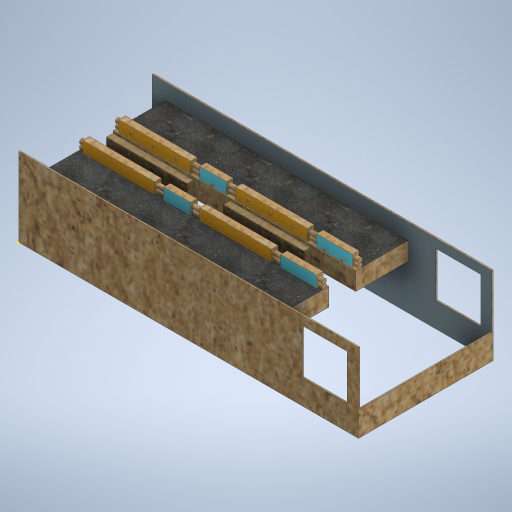
# Autodesk Inventor part: Walls
Saved by Autodesk Inventor 2024 (Build 280153000, 153)
## iProperties
Created: 2024-02-01
Part Number: Walls
Material: Generic
Document SubType Name: Modeling
Designer: HP
Density: 1 g/cm^3
Appearance: Default
Author: HP
Autodesk Inventor part; units mm, degrees
ref_plane "YZ Plane" through (0, 0, 0) normal (1, 0, 0) x (0, 1, 0)
sketch "Sketch2" plane through (0, 0, 0) normal (1, 0, 0) x (0, 1, 0)
  line L0 (0, 0) -> (175, 0)
  line L1 (175, 0) -> (175, 3)
  line L2 (175, 3) -> (0, 3)
  line L3 (0, 3) -> (0, 0)
  line L4 (0, 300) -> (175, 300)
  line L5 (175, 300) -> (175, 297)
  line L6 (175, 297) -> (0, 297)
  line L7 (0, 297) -> (0, 300)
  dimension "d8" = 175
  dimension "d9" = 3
  dimension "d10" = 175
  dimension "d11" = 3
  constraints: 16 end point, 4 parallel, 2 horizontal, 2 perpendicular, 1 point on line
  measures "d8" distance of L2.end L1.end
  measures "d9" distance of L1.end L0.end
  measures "d10" distance of L5.end L6.end
  measures "d11" distance of L4.end L5.end
extrude "Extrusion2" add sketch "Sketch2" along normal blind 756
sketch "Sketch3" plane through (0, 0, 300) normal (0, 0, 1) x (1, 0, 0)
  point P0 (0, 0)
sketch "Sketch4" plane through (0, 0, 300) normal (0, 0, 1) x (1, 0, 0)
  line L0 (0, 0) -> (3, 0)
  line L1 (3, 0) -> (3, 55)
  line L2 (3, 55) -> (0, 55)
  line L3 (0, 55) -> (0, 0)
  line L4 (756, 0) -> (753, 0)
  line L5 (753, 0) -> (753, 55)
  line L6 (753, 55) -> (756, 55)
  line L7 (756, 55) -> (756, 0)
  dimension "d30" = 100
  dimension "d31" = 100
  dimension "d32" = 25
  dimension "d41" = 55
  dimension "d14" = 3
  dimension "d15" = 55
  dimension "d16" = 3
  dimension "d17" = 55
  constraints: 16 end point, 4 parallel, 2 horizontal, 2 perpendicular
  measures "d14" distance of L2.end L1.end
  measures "d15" distance of L1.end L0.end
  measures "d16" distance of L5.end L6.end
  measures "d17" distance of L4.end L5.end
extrude "Extrusion3" add sketch "Sketch4" against normal through all
sketch "Sketch5" plane through (0, 0, 300) normal (0, 0, 1) x (1, 0, 0)
  point P0 (0, 0)
sketch "Sketch6" plane through (0, 0, 300) normal (0, 0, 1) x (1, 0, 0)
  point P0 (0, 0)
sketch "Sketch10" plane through (0, 0, 300) normal (0, 0, 1) x (1, 0, 0)
  line L0 (631, 155) -> (731, 155)
  line L1 (731, 155) -> (731, 55)
  line L2 (731, 55) -> (631, 55)
  line L3 (631, 55) -> (631, 155)
  line L4 (756, 175) -> (756, 0) projected
  line L5 (0, 175) -> (756, 175) projected
  line L6 (0, 0) -> (756, 0) projected
  dimension "d30" = 100
  dimension "d31" = 100
  dimension "d32" = 25
  dimension "d41" = 55
  constraints: 8 end point, 2 parallel, 1 horizontal, 1 perpendicular
  measures "d30" distance of L1.end L2.end
  measures "d31" distance of L0.end L1.end
  measures "d32" distance between parallel lines of L4 L1
  measures "d41" distance between parallel lines of L6 L2
extrude "Extrusion4" cut sketch "Sketch10" against normal through all
sketch "Sketch11" plane through (0, 0, 0) normal (0, -1, 0) x (1, 0, 0)
  point P0 (0, 0)
sketch "Sketch16" plane through (0, 0, 300) normal (0, 0, 1) x (1, 0, 0)
  line L0 (30, 140) -> (570, 140)
  line L1 (570, 140) -> (570, 100)
  line L2 (570, 100) -> (30, 100)
  line L3 (30, 100) -> (30, 140)
  line L4 (0, 175) -> (0, 0) projected
  line L5 (0, 0) -> (756, 0) projected
  point P0 (0, 87.5)
  dimension "d55" = 540
  dimension "d56" = 40
  dimension "d57" = 30
  dimension "d58" = 100
  constraints: 8 end point, 2 parallel, 1 horizontal, 1 midpoint, 1 perpendicular
  measures "d55" distance of L1.end L2.end
  measures "d56" distance of L0.end L1.end
  measures "d57" distance from line of point (0, 87.5) L3
  measures "d58" distance between parallel lines of L5 L2
extrude "Extrusion8" add sketch "Sketch16" against normal blind 120
ref_plane "Work Plane4" through (0, 0, 150) normal (0, 0, 1) x (1, 0, 0)
mirror "Mirror3" about plane through (0, 0, 150) normal (0, 0, 1) of "Extrusion8"
sketch "Sketch17" plane through (0, 0, 180) normal (0, 0, -1) x (-1, 0, 0)
  point P0 (0, 0)
sketch "Sketch19" plane through (0, 0, 180) normal (0, 0, -1) x (-1, 0, 0)
  line L0 (-210, 135) -> (-30, 135)
  line L1 (-30, 135) -> (-30, 105)
  line L2 (-30, 105) -> (-210, 105)
  line L3 (-210, 105) -> (-210, 135)
  line L4 (-570, 140) -> (-30, 140) projected
  line L5 (-30, 140) -> (-30, 100) projected
  point P0 (0, 0)
  dimension "d62" = 180
  dimension "d63" = 30
  dimension "d64" = 5
  dimension "d65" = 0
  constraints: 8 end point, 2 parallel, 1 horizontal, 1 perpendicular
  measures "d62" distance of L1.end L2.end
  measures "d63" distance of L0.end L1.end
  measures "d64" distance between parallel lines of L0 L4
  measures "d65" distance between parallel lines of L5 L1
extrude "Extrusion9" add sketch "Sketch19" along normal blind 15
sketch "Sketch21" plane through (0, 0, 165) normal (0, 0, -1) x (-1, 0, 0)
  circle A0 centre (-200, 127.5) radius 2.5
  line L0 (-210, 105) -> (-210, 135) projected
  line L1 (-210, 135) -> (-30, 135) projected
  circle A1 centre (-120, 127.5) radius 2.5
  circle A2 centre (-80, 127.5) radius 2.5
  circle A3 centre (-40, 127.5) radius 2.5
  line L2 (-30, 140) -> (-30, 100) projected
  circle A4 centre (-160, 127.5) radius 2.5
  line L3 (-30, 120) -> (-210, 120)
  circle A5 centre (-200, 112.5) radius 2.5
  circle A6 centre (-120, 112.5) radius 2.5
  circle A7 centre (-80, 112.5) radius 2.5
  circle A8 centre (-40, 112.5) radius 2.5
  circle A9 centre (-160, 112.5) radius 2.5
  point P0 (0, 0)
  dimension "d74" = 5
  dimension "d75" = 10
  dimension "d76" = 7.5
  dimension "d77" = 5
  dimension "d78" = 5
  dimension "d79" = 5
  dimension "d83" = 10
  dimension "d84" = 40
  dimension "d85" = 40
  dimension "d86" = 5
  dimension "d87" = 40
  dimension "d88" = 7.5
  dimension "d89" = 7.5
  dimension "d90" = 7.5
  dimension "d91" = 7.5
  constraints: 10 centre point, 5 symmetric about line, 2 end point, 2 midpoint, 5 other
  measures "d74" diameter of A0
  measures "d75" distance from line of L0 A0.centre
  measures "d76" distance from line of L1 A0.centre
  measures "d77" diameter of A1
  measures "d78" diameter of A2
  measures "d79" diameter of A3
  measures "d83" horizontal distance of L3.start A3.centre
  measures "d84" distance of A3.centre A2.centre
  measures "d85" distance of A2.centre A1.centre
  measures "d86" diameter of A4
  measures "d87" distance of A1.centre A4.centre
  measures "d88" distance from line of L1 A4.centre
  measures "d89" distance from line of L1 A1.centre
  measures "d90" distance from line of L1 A2.centre
  measures "d91" distance from line of L1 A3.centre
extrude "Extrusion11" cut sketch "Sketch21" against normal blind 3 contours A0 | A1 | A2 | A3 | A4 | A5 | A6 | A7 | A8 | A9
sketch "Sketch20" plane through (0, 0, 180) normal (0, 0, -1) x (-1, 0, 0)
  line L0 (-470, 135) -> (-290, 135)
  line L1 (-290, 135) -> (-290, 105)
  line L2 (-290, 105) -> (-470, 105)
  line L3 (-470, 105) -> (-470, 135)
  line L4 (-570, 140) -> (-30, 140) projected
  line L5 (-30, 140) -> (-30, 100) projected
  point P0 (0, 0)
  dimension "d68" = 180
  dimension "d69" = 30
  dimension "d70" = 5
  dimension "d71" = 260
  constraints: 8 end point, 2 parallel, 1 horizontal, 1 perpendicular
  measures "d68" distance of L1.end L2.end
  measures "d69" distance of L0.end L1.end
  measures "d70" distance between parallel lines of L4 L0
  measures "d71" distance between parallel lines of L5 L1
extrude "Extrusion10" add sketch "Sketch20" along normal blind 15
sketch "Sketch22" plane through (0, 0, 165) normal (0, 0, -1) x (-1, 0, 0)
  circle A0 centre (-460, 127.5) radius 2.5
  circle A1 centre (-420, 127.5) radius 2.5
  circle A2 centre (-380, 127.5) radius 2.5
  circle A3 centre (-340, 127.5) radius 2.5
  circle A4 centre (-300, 127.5) radius 2.5
  line L0 (-470, 135) -> (-290, 135) projected
  line L1 (-470, 105) -> (-470, 135) projected
  line L2 (-470, 120) -> (-290, 120)
  line L3 (-290, 135) -> (-290, 105) projected
  circle A5 centre (-460, 112.5) radius 2.5
  circle A6 centre (-420, 112.5) radius 2.5
  circle A7 centre (-380, 112.5) radius 2.5
  circle A8 centre (-340, 112.5) radius 2.5
  circle A9 centre (-300, 112.5) radius 2.5
  point P0 (0, 0)
  dimension "d94" = 5
  dimension "d95" = 5
  dimension "d96" = 5
  dimension "d97" = 5
  dimension "d98" = 5
  dimension "d99" = 7.5
  dimension "d100" = 7.5
  dimension "d101" = 7.5
  dimension "d102" = 7.5
  dimension "d103" = 10
  dimension "d104" = 40
  dimension "d105" = 40
  dimension "d106" = 40
  dimension "d107" = 40
  dimension "d108" = 7.5
  constraints: 10 centre point, 5 symmetric about line, 2 end point, 2 midpoint, 5 other
  measures "d94" diameter of A0
  measures "d95" diameter of A1
  measures "d96" diameter of A2
  measures "d97" diameter of A3
  measures "d98" diameter of A4
  measures "d99" distance from line of L0 A0.centre
  measures "d100" distance from line of L0 A1.centre
  measures "d101" distance from line of L0 A2.centre
  measures "d102" distance from line of L0 A3.centre
  measures "d103" distance from line of L1 A0.centre
  measures "d104" distance of A0.centre A1.centre
  measures "d105" distance of A1.centre A2.centre
  measures "d106" distance of A2.centre A3.centre
  measures "d107" distance of A4.centre A3.centre
  measures "d108" distance from line of L0 A4.centre
extrude "Extrusion12" cut sketch "Sketch22" against normal blind 3 contours A0 | A1 | A2 | A3 | A4 | A5 | A6 | A7 | A8 | A9
ref_plane "Work Plane5" through (0, 0, 150) normal (0, 0, 1) x (1, 0, 0)
mirror "Mirror4" about plane through (0, 0, 150) normal (0, 0, 1) of "Extrusion8", "Extrusion9", "Extrusion10", "Extrusion12", "Extrusion11"
sketch "Sketch23" plane through (570, 100, 3) normal (1, 0, 0) x (0, 0, -1)
  circle A0 centre (-107, 45) radius 5
  circle A1 centre (-107, 55) radius 5
  line L0 (0, 40) -> (-117, 40) projected
  line L1 (-117, 40) -> (-117, 0) projected
  point P0 (3, -100)
  point P1 (-107, 50)
  dimension "d112" = 10
  dimension "d113" = 10
  dimension "d114" = 5
  dimension "d115" = 10
  dimension "d116" = 0
  dimension "d117" = 10
  constraints: 2 centre point
  measures "d112" diameter of A0
  measures "d113" diameter of A1
  measures "d114" distance from line of L0 A0.centre
  measures "d115" distance of A0.centre A1.centre
  measures "d116" horizontal distance of A1.centre A0.centre
  measures "d117" distance from line of A0.centre L1
extrude "Extrusion13" add sketch "Sketch23" against normal blind 540
sketch "Sketch24" plane through (30, 140, 3) normal (0, 1, 0) x (1, 0, 0)
  line L0 (450, -114.5) -> (530, -114.5)
  line L1 (530, -114.5) -> (530, -99.5)
  line L2 (530, -99.5) -> (450, -99.5)
  line L3 (450, -99.5) -> (450, -114.5)
  line L4 (0, -117) -> (540, -117) projected
  line L5 (440, -117) -> (440, -132) projected
  point P0 (-30, 3)
  dimension "d120" = 80
  dimension "d121" = 15
  dimension "d122" = 2.5
  dimension "d123" = 10
  constraints: 8 end point, 2 parallel, 1 horizontal, 1 perpendicular
  measures "d120" distance of L2.end L1.end
  measures "d121" distance between parallel lines of L0 L2
  measures "d122" distance between parallel lines of L4 L0
  measures "d123" distance between parallel lines of L5 L3
extrude "Extrusion14" add sketch "Sketch24" along normal blind 25
sketch "Sketch25" plane through (30, 140, 3) normal (0, 1, 0) x (1, 0, 0)
  line L0 (270, -99.5) -> (430, -99.5)
  line L1 (430, -99.5) -> (430, -114.5)
  line L2 (430, -114.5) -> (270, -114.5)
  line L3 (270, -114.5) -> (270, -99.5)
  line L4 (0, -117) -> (540, -117) projected
  line L5 (260, -117) -> (260, -132) projected
  point P0 (-30, 3)
  dimension "d126" = 160
  dimension "d127" = 15
  dimension "d128" = 17.5
  dimension "d129" = 10
  constraints: 8 end point, 2 parallel, 1 horizontal, 1 perpendicular
  measures "d126" distance of L1.end L2.end
  measures "d127" distance of L0.end L1.end
  measures "d128" distance between parallel lines of L4 L0
  measures "d129" distance between parallel lines of L5 L3
extrude "Extrusion15" add sketch "Sketch25" along normal blind 25
sketch "Sketch26" plane through (30, 140, 3) normal (0, 1, 0) x (1, 0, 0)
  line L0 (190, -99.5) -> (250, -99.5)
  line L1 (250, -99.5) -> (250, -114.5)
  line L2 (250, -114.5) -> (190, -114.5)
  line L3 (190, -114.5) -> (190, -99.5)
  line L4 (0, -117) -> (540, -117) projected
  line L5 (180, -117) -> (180, -132) projected
  line L6 (10, -99.5) -> (170, -99.5)
  line L7 (170, -99.5) -> (170, -114.5)
  line L8 (170, -114.5) -> (10, -114.5)
  line L9 (10, -114.5) -> (10, -99.5)
  line L10 (0, -102) -> (0, -112) projected
  point P0 (-30, 3)
  point P1 (0, -107)
  dimension "d132" = 60
  dimension "d133" = 15
  dimension "d134" = 17.5
  dimension "d135" = 10
  dimension "d136" = 160
  dimension "d137" = 15
  dimension "d138" = 17.5
  dimension "d139" = 10
  constraints: 16 end point, 4 parallel, 2 horizontal, 2 perpendicular
  measures "d132" distance of L1.end L2.end
  measures "d133" distance of L0.end L1.end
  measures "d134" distance between parallel lines of L4 L0
  measures "d135" distance between parallel lines of L5 L3
  measures "d136" distance of L7.end L8.end
  measures "d137" distance of L6.end L7.end
  measures "d138" distance between parallel lines of L4 L6
  measures "d139" distance between parallel lines of L10 L9
extrude "Extrusion16" add sketch "Sketch26" along normal blind 25
sketch "Sketch27" plane through (480, 140, 117.5) normal (0, 0, 1) x (1, 0, 0)
  circle A0 centre (-50, 15) radius 2.5
  circle A1 centre (-100, 15) radius 2.5
  circle A2 centre (-150, 15) radius 2.5
  circle A3 centre (-310, 15) radius 2.5
  circle A4 centre (-360, 15) radius 2.5
  circle A5 centre (-410, 15) radius 2.5
  line L0 (-440, 20) -> (-440, 10) projected
  line L1 (-280, 10) -> (-280, 20) projected
  line L2 (-280, 25) -> (-440, 25) projected
  line L3 (-200, 10) -> (-200, 20) projected
  line L4 (-200, 25) -> (-260, 25) projected
  line L5 (-180, 20) -> (-180, 10) projected
  line L6 (-20, 25) -> (-180, 25) projected
  line L7 (0, 20) -> (0, 10) projected
  line L8 (80, 10) -> (80, 20) projected
  line L9 (80, 25) -> (0, 25) projected
  line L10 (80, 10) -> (-440, 10)
  circle A6 centre (60, 5) radius 2.5
  circle A7 centre (20, 5) radius 2.5
  circle A8 centre (-230, 5) radius 2.5
  point P0 (-480, -140)
  point P1 (-360, 25)
  dimension "d144" = 5
  dimension "d145" = 5
  dimension "d146" = 5
  dimension "d148" = 5
  dimension "d149" = 5
  dimension "d150" = 5
  dimension "d151" = 30
  dimension "d152" = 30
  dimension "d153" = 50
  dimension "d154" = 10
  dimension "d155" = 10
  dimension "d156" = 10
  dimension "d159" = 30
  dimension "d160" = 10
  dimension "d161" = 50
  dimension "d162" = 10
  dimension "d163" = 10
  dimension "d164" = 50
  constraints: 9 centre point, 2 end point, 1 midpoint, 1 perpendicular
  measures "d144" diameter of A0
  measures "d145" diameter of A1
  measures "d146" diameter of A2
  measures "d148" diameter of A3
  measures "d149" diameter of A4
  measures "d150" diameter of A5
  measures "d151" distance from line of A5.centre L0
  measures "d152" distance from line of L1 A3.centre
  measures "d153" distance of A3.centre A4.centre
  measures "d154" distance of point (-360, 25) A4.centre
  measures "d155" distance from line of A5.centre L2
  measures "d156" distance from line of L2 A3.centre
  measures "d159" distance from line of L5 A2.centre
  measures "d160" distance from line of L6 A2.centre
  measures "d161" distance of A2.centre A1.centre
  measures "d162" distance from line of L6 A1.centre
  measures "d163" distance from line of L6 A0.centre
  measures "d164" distance of A1.centre A0.centre
extrude "Extrusion17" add sketch "Sketch27" along normal blind 3
mirror "Mirror5" about plane through (0, 0, 150) normal (0, 0, 1) of "Extrusion16", "Extrusion15", "Extrusion13", "Extrusion17", "Extrusion14"
body "Solid2"
